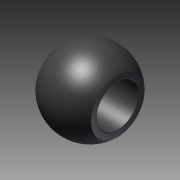
# Autodesk Inventor part: POS 12 Ball
Saved by Autodesk Inventor 2011 SP1 (Build 150282100, 282)
## iProperties
Created: 2017-09-12
Part Number: POS 12 Ball
Catalog Web Link: www.cadenas.de
Description: rod end with male thread B-
Vendor: IKO
Document SubType Name: Modeling
Designer: psAdmin
Manufacturer: IKO
Mass: 3.31082 g
Surface Area: 18.5864 cm^2
Volume: 3.31082 cm^3
Density: 1 g/cm^3
Category: PARTsolutions
Company: IKO
Title: POS 12 Ball
Author: Cadenas PARTsolutions
PSOL_IDENT_0: {$CADENAS_DATA\23d-libs\iko\iko_bearings\pillobals\insert_type\rod_end_with_male_thread_ball.prj},18
PSOL_IDENT_1: 4 {VTYP=3D},{NB=POS 12 Ball},{LINA=POS 12 Ball},{NN=rod end with male thread B},{DATE=13.10.2016 10:
PSOL_IDENT_2: 02:13},{GEOMDATE=02.01.2008 13:56:00},{VERSION=},{LINEID=70},{LINESUBID=-1},{WBVAR=}  {NB=POS 12 Bal
PSOL_IDENT_3: l},{LINA=POS 12 Ball},{KT=DUMMY},{IDNR=},{RID=G_70},{STDRT=12},{DESCR=(gevmsg IKOSTV 914)},{TRNUMBER=
PSOL_IDENT_4: },{PAST=A},{REST=O},{ORDER=POS 12},{MASS=85.0},{SD=12},{G=M12x1.75},{P1=1.750},{NDM=12.000},{SD2=30}
PSOL_IDENT_5: ,{C1=12.0},{B=16},{SD1=15.4},{SL2=69},{SH=54},{SL1=33},{SR1=0.2},{DBL=22.23},{C2=0.00},{C3=0.00},{AA=
PSOL_IDENT_6: 0.00},{BB=0},{R2=3.0},{R3=22.5},{H2=41.03},{CGN=4.5},{P=2.5},{C=60},{LL6=34.56},{LL7=0.00},{LL8=2.34
PSOL_IDENT_7: },{LL9=0.00},{LL10=0.00},{CD=13100},{CS=16900},{G1=12},{GG1=10.11},{PP=1.8},{ALFA=55},{BL=4},{SC=1}
NN: rod end with male thread B
NB: POS 12 Ball
NBSYN: $ORDER. Ball
LINA: POS 12 Ball
RID: G_70
STDRT: 12
DESCR: (gevmsg IKOSTV 914)
PAST: A
REST: O
ORDER: POS 12
MASS: 85.0
SD: 12
G: M12x1.75
P1: 1.750
NDM: 12.000
SD2: 30
C1: 12.0
B: 16
SD1: 15.4
SL2: 69
SH: 54
SL1: 33
SR1: 0.2
DBL: 22.23
C2: 0.00
C3: 0.00
AA: 0.00
BB: 0
R2: 3.0
R3: 22.5
H2: 41.03
CGN: 4.5
P: 2.5
C: 60
LL6: 34.56
LL7: 0.00
LL8: 2.34
LL9: 0.00
LL10: 0.00
CD: 13100
CS: 16900
G1: 12
GG1: 10.11
PP: 1.8
ALFA: 55
BL: 4
SC: 1
SUPPLIER: IKO
ARTICLENO: POS 12 Ball
BOMINFO: POS 12 Ball
CREATOR: CADENAS GmbH
Autodesk Inventor part; units mm, degrees
sketch "Sketch_1" plane through (0, 0, 0) normal (0, 0, 1) x (1, 0, 0)
  line L0 (16, 0) -> (0, 0)
  arc A0 (0, 6.2) -> (0.2, 6) centre (0.2, 6.2) ccw
  line L1 (0.2, 6) -> (15.8, 6)
  arc A1 (15.8, 6) -> (16, 6.2) centre (15.8, 6.2) ccw
  line L2 (16, 6.2) -> (16, 7.7)
  arc A2 (16, 7.7) -> (0, 7.7) centre (8, -0.0164) ccw
  line L3 (0, 7.7) -> (0, 6.2)
  constraints: 8 end point, 6 point on circle, 3 centre point
revolve "Revolution1" add sketch "Sketch_1" angle 360 about axis through (16, 0, 0) along (1, 0, 0)
ref_plane "IP1_XY" through (8, 0, 0) normal (-1, 0, 0) x (0, 0, -1)
ref_plane "IP1_YZ" through (8, 0, 0) normal (0, 0, -1) x (0, -1, 0)
ref_plane "IP1_ZX" through (8, 0, 0) normal (0, -1, 0) x (-1, 0, 0)
body "Solid1"
